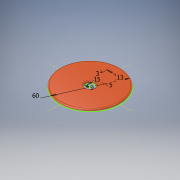
# Autodesk Inventor part: Stewart-Plate-Head
Saved by Autodesk Inventor 2018.2 (Build 222227000, 227)
## iProperties
Created: 2018-02-18
Part Number: Stewart-Plate-Head
Material: Generisch
Document SubType Name: Modeling
Designer: JochenAlt
Density: 1 g/cm^3
Appearance: Vorgabe
Author: JochenAlt
Autodesk Inventor part; units mm, degrees
ref_plane "YZ Plane" through (0, 0, 0) normal (1, 0, 0) x (0, 1, 0)
ref_plane "XZ Plane" through (0, 0, 0) normal (0, 1, 0) x (-1, 0, 0)
ref_plane "XY Plane" through (0, 0, 0) normal (0, 0, 1) x (1, 0, 0)
sketch "Skizze1" plane through (0, 0, 0) normal (0, 0, 1) x (1, 0, 0)
  line L0 (-42, 0) -> (42, 0) construction
  circle A0 centre (0, 0) radius 30
  line L1 (-6.5, 18) -> (6.5, 18)
  line L2 (6.5, 18) -> (6.5, 15)
  line L3 (6.5, 15) -> (-6.5, 15)
  line L4 (-6.5, 15) -> (-6.5, 18)
  line L5 (1.5, 15) -> (-1.5, 15)
  line L6 (-1.5, 15) -> (-1.5, 10)
  line L7 (-1.5, 10) -> (1.5, 10)
  line L8 (1.5, 10) -> (1.5, 15)
  circle A1 centre (0, 0) radius 4.5
  line L9 (0, 42) -> (0, -42) construction
  dimension "d9" = 60
  dimension "d10" = 3
  dimension "d11" = 15
  dimension "d14" = 13
  dimension "d23" = 5
  dimension "d62" = 9
  constraints: 16 end point, 4 parallel, 3 perpendicular, 2 centre point, 2 horizontal, 1 coincident, 1 midpoint, 1 point on line, 1 other
  measures "d9" diameter of A0
  measures "d10" distance between parallel lines of L3 L1
  measures "d11" distance from line of L3 A0.centre
  measures "d14" distance between parallel lines of L2 L4
  measures "d23" distance between parallel lines of L3 L7
  measures "d62" diameter of A1
extrude "Extrusion3" add sketch "Skizze1" against normal blind 7 contours L1 L2 L3 L4 | L3 L8 L7 L6
fillet "Rundung1" radius 4 2 edges at (-6.5, 16.5, -7) (6.5, 16.5, -7)
sketch "Skizze2" plane through (-6.5, 18, 0) normal (0, 1, 0) x (1, 0, 0)
  circle A0 centre (3, 4) radius 1.1
  circle A1 centre (10, 4) radius 1.1
  line L0 (6.5, 0) -> (6.5, 7) construction
  line L1 (43, 0) -> (-27, 0) construction
  line L2 (-1.6221, 4) -> (19.0112, 4) construction
  line L3 (4, 7) -> (9, 7) construction
  line L4 (0, 0) -> (0, 3) projected
  dimension "d16" = 2.2
  dimension "d20" = 3
  dimension "d21" = 3
  constraints: 4 end point, 2 centre point, 1 equal radius, 1 horizontal, 1 midpoint, 1 point on line, 1 symmetric about line, 1 vertical
  measures "d16" diameter of A0
  measures "d20" distance between parallel lines of L3 L2
  measures "d21" distance from line of L4 A0.centre
extrude "Extrusion4" cut sketch "Skizze2" against normal up to next
chamfer "Fase1" distance 5 distance2 7 1 edges at (0, 10, -7) measured on face at (0, 10.5, -7)
pattern_circular "Runde Anordnung1" count 3 over 360 about axis through (0, 0, -10) along (0, 0, 1) of "Extrusion3", "Extrusion4", "Fase1", "Rundung1"
extrude "Extrusion11" add sketch "Skizze1" along normal blind 2 contours A0 | L1 L2 L3 L4 | L3 L8 L7 L6
fillet "Rundung5" radius 1 4 edges at (-30, 0, 2) (-4.5, 0, 2) (-4.5, 0, 0) (-30, 0, 0)
equation "\"d21\" = d20"
